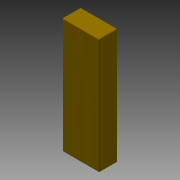
# Autodesk Inventor part: Battery
Saved by Autodesk Inventor 2015 (Build 190159000, 159)
## iProperties
Created: 2015-10-20
Part Number: Battery
Material: Generic
Document SubType Name: Modeling
Designer: James
Density: 1 g/cm^3
Appearance: Default
Author: James
Autodesk Inventor part; units mm, degrees
ref_plane "YZ Plane" through (0, 0, 0) normal (1, 0, 0) x (0, 1, 0)
ref_plane "XZ Plane" through (0, 0, 0) normal (0, 1, 0) x (-1, 0, 0)
ref_plane "XY Plane" through (0, 0, 0) normal (0, 0, 1) x (1, 0, 0)
sketch "Sketch1" plane through (0, 0, 0) normal (0, 1, 0) x (-1, 0, 0)
  line L0 (-17, 53) -> (-17, -53)
  line L1 (-17, -53) -> (17, -53)
  line L2 (17, -53) -> (17, 53)
  line L3 (17, 53) -> (-17, 53)
  line L4 (-17, 53) -> (17, -53) construction
  line L5 (-17, -53) -> (17, 53) construction
  point P0 (0, 0)
  dimension "d0" = 106
  dimension "d1" = 34
  constraints: 12 end point, 2 midpoint, 2 parallel, 1 perpendicular, 1 vertical
  measures "d0" distance of L0.start L0.end
  measures "d1" distance of L1.end L0.end
extrude "Extrusion1" add sketch "Sketch1" along normal blind 17
fillet "Fillet1" radius 1 12 edges at (17, 17, 0) (0, 17, 53) (17, 8.5, 53) (17, 0, 0) (17, 8.5, -53) (0, 17, -53) (-17, 17, 0) (-17, 8.5, 53) (0, 0, 53) (-17, 0, 0) (-17, 8.5, -53) (0, 0, -53)
body "Solid1"
